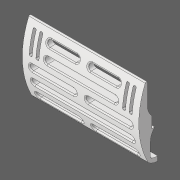
# Autodesk Inventor part: HandPlate1_Center
Saved by Autodesk Inventor 2020 (Build 240168000, 168)
## iProperties
Created: 2020-01-12
Part Number: HandPlate1_Center
Material: PLA Plastic (Black)
Document SubType Name: Modeling
Designer: Isaac Newcomb
Density: 1 g/cm^3
Appearance: 3D Printed - Black
Mass: 114.76 g
Surface Area: 433.989 cm^2
Volume: 114.76 cm^3
Author: Isaac Newcomb
Autodesk Inventor part; units mm, degrees
ref_plane "YZ Plane" through (0, 0, 0) normal (1, 0, 0) x (0, 1, 0)
ref_plane "XZ Plane" through (0, 0, 0) normal (0, 1, 0) x (-1, 0, 0)
ref_plane "XY Plane" through (0, 0, 0) normal (0, 0, 1) x (1, 0, 0)
sketch "Profile" plane through (0, 0, 0) normal (0, 0, 1) x (1, 0, 0)
  arc A0 (-13.7625, 56.5) -> (-16.6445, 57.0832) centre (-15.2625, 56.5) ccw
  line L0 (-7.7625, 0) -> (-7.7625, 15)
  arc A1 (-13.7625, 29.2829) -> (-7.7625, 15) centre (6.2375, 29.2829) ccw
  arc A2 (-16.6445, 57.0832) -> (-12.8608, -36.4892) centre (84.7024, 14.3185) ccw
  line L1 (0, 0) -> (-7.7625, 0)
  line L2 (-13.7625, 56.5) -> (-13.7625, 29.2829)
  line L3 (0, -41.5035) -> (0, -35.5035)
  line L4 (0, -35.5035) -> (-7.7625, -35.5035) construction
  arc A3 (-12.8608, -36.4892) -> (-12, -37.5035) centre (-10.2, -35.1035) ccw
  arc A4 (-9.8812, -31.3441) -> (-7.8643, -34.1785) centre (-6.8812, -31.3441) ccw
  arc A5 (-12, -37.5035) -> (0, -41.5035) centre (0, -21.5035) ccw
  line L5 (0, -41.5035) -> (-7.7625, -41.5035) construction
  arc A6 (-7.8643, -34.1785) -> (0, -35.5035) centre (0, -11.5035) ccw
  line L6 (-9.8812, -14.2829) -> (-9.8812, -31.3441)
  arc A7 (-3.8812, 0) -> (-9.8812, -14.2829) centre (10.1188, -14.2829) ccw
  dimension "height" = 56.5
  dimension "d3" = 1.5
  dimension "d5" = 15
  dimension "d100" = 110
  dimension "d114" = 20
  dimension "d115" = 7.7625
  dimension "d122" = 6
  dimension "d124" = 6
  dimension "d127" = 3
  dimension "d129" = 20
  dimension "d130" = 41.5035
  dimension "d131" = 12
  dimension "d133" = 20
  dimension "d134" = 6
  dimension "d135" = 3
  dimension "d136" = 10
  constraints: 17 point on circle, 14 end point, 10 tangent, 8 centre point, 4 vertical, 3 point on line, 2 midpoint, 2 perpendicular, 1 horizontal
  measures "height" vertical distance of A0.centre L1.start
  measures "d3" radius of A0
  measures "d5" distance of L0.start L0.end
  measures "d100" radius of A2
  measures "d114" radius of A1
  measures "d115" distance from line of L0 L1.start
  measures "d122" distance from line of L0 L2.start
  measures "d124" distance of L3.start L3.end
  measures "d127" radius of A3
  measures "d129" radius of A5
  measures "d130" distance of L1.start L3.start
  measures "d131" horizontal distance of L3.start A3.end
  measures "d133" radius of A7
  measures "d134" distance from line of A7.start L6
  measures "d135" radius of A4
  measures "d136" distance of A6.centre A5.centre
extrude "Extrusion" add sketch "Profile" along normal blind 156
sketch "Slot Sketch" plane through (0, 0, 0) normal (0, 1, 0) x (-1, 0, 0)
  line L0 (7.7625, 79.5) -> (10.7625, 81) construction
  line L1 (10.7625, 81) -> (10.7625, 75) construction
  line L2 (10.7625, 75) -> (7.7625, 76.5) construction
  line L3 (7.7625, 76.5) -> (7.7625, 79.5)
  line L4 (7.7625, 78) -> (11.0625, 78) construction
  line L5 (7.7625, 76.5) -> (7.7625, 76.1646)
  line L6 (7.7625, 76.1646) -> (11.0625, 74.5146)
  line L7 (11.0625, 74.5146) -> (11.0625, 81.4854)
  line L8 (11.0625, 81.4854) -> (7.7625, 79.8354)
  line L9 (7.7625, 79.8354) -> (7.7625, 79.5)
  point P0 (0, 0)
  point P1 (10.7625, 78)
  dimension "d36" = 0.3
  dimension "d37" = 0.3
  dimension "d38" = 3
  dimension "d39" = 6
  dimension "d40" = 3
  dimension "d141" = 7.7625
  dimension "d142" = 78
  constraints: 20 end point, 3 midpoint, 3 vertical, 2 parallel, 2 point on line, 1 collinear, 1 horizontal
  measures "d36" distance between parallel lines of L7 L1
  measures "d37" distance between parallel lines of L0 L8
  measures "d38" distance between parallel lines of L3 L1
  measures "d39" distance of L0.end L2.start
  measures "d40" distance of L2.end L3.end
  measures "d141" distance from line of point (0, 0) L3
  measures "d142" distance from line of point (0, 0) L4
extrude "Mounting Slots" cut sketch "Slot Sketch" along normal through all
sketch "Strap Slot Sketch" plane through (0, 0, 0) normal (1, 0, 0) x (0, 1, 0)
  line L0 (50, 147) -> (20, 147)
  line L1 (20, 147) -> (20, 143)
  line L2 (20, 143) -> (50, 143)
  line L3 (50, 143) -> (50, 147)
  line L4 (50, 13) -> (20, 13)
  line L5 (20, 13) -> (20, 9)
  line L6 (20, 9) -> (50, 9)
  line L7 (50, 9) -> (50, 13)
  line L8 (35, 13) -> (35, 143) construction
  line L9 (20, 22) -> (50, 22)
  line L10 (50, 22) -> (50, 18)
  line L11 (50, 18) -> (20, 18)
  line L12 (20, 18) -> (20, 22)
  line L13 (20, 138) -> (50, 138)
  line L14 (50, 138) -> (50, 134)
  line L15 (50, 134) -> (20, 134)
  line L16 (20, 134) -> (20, 138)
  point P0 (0, 0)
  point P1 (35, 78)
  dimension "d48" = 78
  dimension "d50" = 20
  dimension "d51" = 30
  dimension "d52" = 4
  dimension "d56" = 5
  dimension "d57" = 5
  dimension "d137" = 120
  constraints: 34 end point, 8 parallel, 5 collinear, 4 horizontal, 4 perpendicular, 4 point on line, 3 midpoint
  measures "d48" vertical distance of point (0, 0) point (35, 78)
  measures "d50" distance from line of L5 point (0, 0)
  measures "d51" distance of L5.end L6.end
  measures "d52" distance of L6.end L4.start
  measures "d56" distance between parallel lines of L2 L13
  measures "d57" distance between parallel lines of L4 L11
  measures "d137" distance between parallel lines of L13 L11
extrude "Strap Slots" cut sketch "Strap Slot Sketch" against normal through all
fillet "Strap Slot Fillet" radius 1.5 16 edges at (-16.5561, 50, 13) (-18.3143, 20, 13) (-18.3143, 20, 9) (-16.5561, 50, 9) (-16.5561, 50, 138) (-18.3143, 20, 138) (-18.3143, 20, 134) (-16.5561, 50, 134) (-18.3143, 20, 143) (-16.5561, 50, 143) (-18.3143, 20, 147) (-16.5561, 50, 147) (-16.5561, 50, 22) (-16.5561, 50, 18) (-18.3143, 20, 18) (-18.3143, 20, 22)
sketch "Cosmetic Slot Sketch" plane through (0, 0, 0) normal (1, 0, 0) x (0, 1, 0)
  line L0 (25.5, 123) -> (25.5, 33) construction
  line L1 (21.5, 123) -> (21.5, 33)
  line L2 (29.5, 33) -> (29.5, 123)
  arc A0 (29.5, 123) -> (21.5, 123) centre (25.5, 123) ccw
  arc A1 (21.5, 33) -> (29.5, 33) centre (25.5, 33) ccw
  line L3 (25.5, 78) -> (21.5, 78) construction
  line L4 (-10.5, 143) -> (-10.5, 13) construction
  line L5 (-14.5, 143) -> (-14.5, 13)
  line L6 (-6.5, 13) -> (-6.5, 143)
  arc A2 (-6.5, 143) -> (-14.5, 143) centre (-10.5, 143) ccw
  arc A3 (-14.5, 13) -> (-6.5, 13) centre (-10.5, 13) ccw
  line L7 (7.5, 143) -> (7.5, 88) construction
  line L8 (3.5, 143) -> (3.5, 88)
  line L9 (11.5, 88) -> (11.5, 143)
  arc A4 (11.5, 143) -> (3.5, 143) centre (7.5, 143) ccw
  arc A5 (3.5, 88) -> (11.5, 88) centre (7.5, 88) ccw
  line L10 (7.5, 68) -> (7.5, 13) construction
  line L11 (3.5, 68) -> (3.5, 13)
  line L12 (11.5, 13) -> (11.5, 68)
  arc A6 (11.5, 68) -> (3.5, 68) centre (7.5, 68) ccw
  arc A7 (3.5, 13) -> (11.5, 13) centre (7.5, 13) ccw
  line L13 (7.5, 68) -> (7.5, 88) construction
  line L14 (-28.5, 68) -> (-28.5, 13) construction
  line L15 (-32.5, 68) -> (-32.5, 13)
  line L16 (-24.5, 13) -> (-24.5, 68)
  arc A8 (-24.5, 68) -> (-32.5, 68) centre (-28.5, 68) ccw
  arc A9 (-32.5, 13) -> (-24.5, 13) centre (-28.5, 13) ccw
  line L17 (-28.5, 143) -> (-28.5, 88) construction
  line L18 (-32.5, 143) -> (-32.5, 88)
  line L19 (-24.5, 88) -> (-24.5, 143)
  arc A10 (-24.5, 143) -> (-32.5, 143) centre (-28.5, 143) ccw
  arc A11 (-32.5, 88) -> (-24.5, 88) centre (-28.5, 88) ccw
  line L20 (-28.5, 88) -> (-28.5, 68) construction
  line L21 (43.5, 123) -> (43.5, 88) construction
  line L22 (39.5, 123) -> (39.5, 88)
  line L23 (47.5, 88) -> (47.5, 123)
  arc A12 (47.5, 123) -> (39.5, 123) centre (43.5, 123) ccw
  arc A13 (39.5, 88) -> (47.5, 88) centre (43.5, 88) ccw
  line L24 (43.5, 68) -> (43.5, 33) construction
  line L25 (39.5, 68) -> (39.5, 33)
  line L26 (47.5, 33) -> (47.5, 68)
  arc A14 (47.5, 68) -> (39.5, 68) centre (43.5, 68) ccw
  arc A15 (39.5, 33) -> (47.5, 33) centre (43.5, 33) ccw
  line L27 (43.5, 68) -> (43.5, 88) construction
  line L28 (25.5, 123) -> (43.5, 123) construction
  line L29 (43.5, 33) -> (25.5, 33) construction
  line L30 (-28.5, 13) -> (7.5, 13) construction
  point P0 (0, 0)
  point P1 (-10.5, 78)
  point P2 (7.5, 115.5)
  point P3 (7.5, 40.5)
  point P4 (7.5, 78)
  point P5 (-28.5, 40.5)
  point P6 (-28.5, 115.5)
  point P7 (-28.5, 78)
  point P8 (43.5, 105.5)
  point P9 (43.5, 50.5)
  point P10 (43.5, 78)
  dimension "d83" = 78
  dimension "d85" = 7.5
  dimension "d88" = 10
  dimension "d89" = 10
  dimension "d95" = 10
  dimension "d98" = 90
  dimension "d99" = 10
  dimension "d138" = 130
  dimension "d139" = 20
  dimension "d140" = 4
  constraints: 78 end point, 32 point on circle, 32 tangent, 16 centre point, 13 midpoint, 10 point on line, 9 parallel, 8 vertical, 7 equal radius, 5 equal length, 3 horizontal
  measures "d83" distance from line of point (0, 0) L3
  measures "d85" distance from line of point (0, 0) L10
  measures "d88" distance between parallel lines of L8 L6
  measures "d89" distance between parallel lines of L1 L9
  measures "d95" distance between parallel lines of L5 L19
  measures "d98" distance of L21.start L24.end
  measures "d99" distance between parallel lines of L2 L22
  measures "d138" distance of L17.start L14.end
  measures "d139" distance of L24.start L21.end
  measures "d140" radius of A15
extrude "Cosmetic Slots" cut sketch "Cosmetic Slot Sketch" against normal through all
fillet "Cosmetic Slot Fillet" radius 1.5 32 edges at (-21.3501, 43.5225, 29.0001) (-20.1737, 47.5, 50.5) (-21.3539, 43.5086, 72) (-22.3766, 39.5, 50.5) (-20.1737, 47.5, 105.5) (-21.3539, 43.5086, 127) (-22.3766, 39.5, 105.5) (-21.3501, 43.5225, 84.0001) (-24.7318, 25.4613, 126.9998) (-25.063, 21.5, 78) (-24.7275, 25.5033, 29) (-24.245, 29.5, 78) (-25.2615, 11.5, 115.5) (-25.0823, 7.4398, 146.9995) (-24.7643, 3.5, 115.5) (-25.0855, 7.4896, 84) (-25.0855, 7.4896, 9) (-25.2615, 11.5, 40.5) (-25.0823, 7.4398, 71.9995) (-24.7643, 3.5, 40.5) (-22.4558, -10.5234, 9.0001) (-23.3096, -6.5, 78) (-22.4455, -10.568, 146.9994) (-21.4555, -14.5, 78) (-16.6086, -28.531, 9.0001) (-18.2205, -24.5, 40.5) (-16.6083, -28.5317, 71.9999) (-14.8367, -32.5, 40.5) (-16.6104, -28.5268, 146.9999) (-14.8367, -32.5, 115.5) (-16.6054, -28.5387, 84.0002) (-18.2205, -24.5, 115.5)
equation "\"d5\" = boxWidth"
equation "\"tabTol\" = 0.3"
equation "\"d14\" = tabTol"
equation "\"d15\" = tabTol"
equation "\"d16\" = bigTabHeight"
equation "\"d17\" = bigTabTopWidth"
equation "\"d18\" = bigTabBaseWidth"
equation "\"d31\" = 0.2"
equation "\"d41\" = 0.2"
equation "\"boxWidth\" = 15"
equation "\"bigTabHeight\" = 3"
equation "\"bigTabTopWidth\" = 6"
equation "\"bigTabBaseWidth\" = 3"
body "Solid1"
